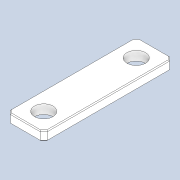
# Autodesk Inventor part: link_c
Saved by Autodesk Inventor 2021 (Build 250183000, 183)
## iProperties
Created: 2020-05-02
Part Number: link_c
Material: Aluminium 6082 T6
Document SubType Name: Modeling
Designer: Hannah
Density: 2.7 g/cm^3
Appearance: Aluminum - Dark
Mass: 16.5538 g
Surface Area: 35.5719 cm^2
Volume: 6.13105 cm^3
Vendor: Custom
Description: seatpost clamp link
Author: Hannah
Revision Number: 1
Autodesk Inventor part; units mm, degrees
ref_plane "YZ Plane" through (0, 0, 0) normal (1, 0, 0) x (0, 1, 0)
ref_plane "XZ Plane" through (0, 0, 0) normal (0, 1, 0) x (-1, 0, 0)
ref_plane "XY Plane" through (0, 0, 0) normal (0, 0, 1) x (1, 0, 0)
sketch "Sketch1" plane through (0, 0, 0) normal (0, 1, 0) x (-1, 0, 0)
  circle A0 centre (0, 25) radius 5
  circle A1 centre (0, -25) radius 5
  line L0 (10, 35) -> (10, -35)
  line L1 (-10, -35) -> (-10, 35)
  line L2 (10, -35) -> (-10, -35)
  line L3 (10, 35) -> (-10, 35)
  line L4 (0, -25) -> (0, 25) construction
  point P0 (0, 0)
  point P1 (10, 0)
  point P2 (0, -35)
  point P3 (0, 35)
  point P4 (0, 0)
  dimension "d1" = 10
  dimension "d5" = 20
  dimension "d6" = 10
  dimension "d7" = 50
  constraints: 10 end point, 4 midpoint, 3 vertical, 3 vertical alignment, 2 centre point, 2 horizontal, 1 coincident, 1 equal radius, 1 horizontal alignment
  measures "d1" diameter of A0
  measures "d5" distance between parallel lines of L1 L0
  measures "d6" distance from line of L3 L4.end
  measures "d7" distance of L4.start L4.end
extrude "Extrusion1" add sketch "Sketch1" along normal mid plane 5
chamfer "Chamfer1" distance 2 angle 45 4 edges at (10, 0, 35) (-10, 0, 35) (10, 0, -35) (-10, 0, -35)
chamfer "Chamfer2" distance 0.5 angle 45 16 edges at (10, 2.5, 0) (9, 2.5, 34) (0, 2.5, 35) (-9, 2.5, 34) (-10, 2.5, 0) (-9, 2.5, -34) (0, 2.5, -35) (9, 2.5, -34) (9, -2.5, 34) (0, -2.5, 35) (10, -2.5, 0) (-9, -2.5, 34) (-10, -2.5, 0) (-9, -2.5, -34) (0, -2.5, -35) (9, -2.5, -34)
equation "\"d6\" = d5 - d1"
body "Solid1"
